Autodesk Inventor part; units mm, degrees
(part 3 of 3)
sketch "Sketch14" plane through (63, -33.9467, -18.5) normal (0, 0, -1) x (-1, 0, 0)
  line L0 (10.55, 31.8934) -> (35, 31.8934) construction
  line L1 (35, 29.5934) -> (35, 31.8934) construction
  line L2 (32.7, 27.2934) -> (35, 29.5934) construction
  line L3 (7.65, 27.2934) -> (32.7, 27.2934) construction
  line L4 (7.65, 29.4734) -> (7.65, 27.2934) construction
  line L5 (0, 29.4734) -> (7.65, 29.4734) construction
  line L6 (0, 35.2734) -> (0, 29.4734) construction
  line L7 (1.6, 35.2734) -> (0, 35.2734) construction
  line L8 (1.6, 44.1134) -> (1.6, 35.2734) construction
  line L9 (0, 44.1134) -> (1.6, 44.1134) construction
  line L10 (0, 52.9934) -> (0, 44.1134) construction
  line L11 (32.7, 52.9934) -> (0, 52.9934) construction
  line L12 (35, 50.6934) -> (32.7, 52.9934) construction
  line L13 (35, 47.8934) -> (35, 50.6934) construction
  line L14 (35, 47.8934) -> (10.55, 47.8934) construction
  line L15 (10.55, 47.8934) -> (10.55, 31.8934) construction
  circle A0 centre (10.2, 51.4934) radius 0.5 construction
  circle A1 centre (15.2, 51.4934) radius 0.5 construction
  circle A2 centre (20.2, 51.4934) radius 0.5 construction
  circle A3 centre (25.2, 51.4934) radius 0.5 construction
  circle A4 centre (10.2, 28.7934) radius 0.5 construction
  circle A5 centre (12.7, 28.7934) radius 0.5 construction
  circle A6 centre (15.2, 28.7934) radius 0.5 construction
  circle A7 centre (17.7, 28.7934) radius 0.5 construction
  circle A8 centre (20.2, 28.7934) radius 0.5 construction
  circle A9 centre (22.7, 28.7934) radius 0.5 construction
  circle A10 centre (25.2, 28.7934) radius 0.5 construction
  circle A11 centre (27.7, 28.7934) radius 0.5 construction
  circle A12 centre (27.7, 51.4934) radius 0.5 construction
  circle A13 centre (22.7, 51.4934) radius 0.5 construction
  circle A14 centre (17.7, 51.4934) radius 0.5 construction
  circle A15 centre (12.7, 51.4934) radius 0.5 construction
  line L16 (1.6, 43.4784) -> (1.6, 35.9084) construction
  line L17 (0.7, 35.9084) -> (1.6, 35.9084) construction
  line L18 (0.7, 43.4784) -> (0.7, 35.9084) construction
  line L19 (0.7, 43.4784) -> (1.6, 43.4784) construction
  line L20 (28.04, 47.3934) -> (28.04, 44.3934) construction
  line L21 (28.04, 44.3934) -> (29.74, 44.3934) construction
  line L22 (29.74, 44.3934) -> (29.74, 47.3934) construction
  line L23 (29.74, 47.3934) -> (28.04, 47.3934) construction
  line L24 (12.6, 45.8934) -> (12.6, 33.8934) construction
  line L25 (12.6, 33.8934) -> (27.7, 33.8934) construction
  line L26 (27.7, 33.8934) -> (27.7, 45.8934) construction
  line L27 (27.7, 45.8934) -> (12.6, 45.8934) construction
  line L28 (10.55, 47.8934) -> (35.5, 47.8934) construction
  line L29 (35.5, 47.8934) -> (35.5, 31.8934) construction
  line L30 (35.5, 31.8934) -> (10.55, 31.8934) construction
  line L31 (10.55, 31.8934) -> (10.55, 47.8934) construction
  line L32 (12.6, 45.8934) -> (27.7, 45.8934) construction
  line L33 (27.7, 45.8934) -> (27.7, 33.8934) construction
  line L34 (27.7, 33.8934) -> (12.6, 33.8934) construction
  line L35 (12.6, 33.8934) -> (12.6, 45.8934) construction
  line L36 (35, 29.5934) -> (35, 31.8934)
  line L37 (35.5, 31.8934) -> (35, 31.8934)
  line L38 (35.5, 31.8934) -> (35.5, 47.8934)
  line L39 (35.5, 47.8934) -> (35, 47.8934)
  line L40 (35, 47.8934) -> (35, 50.6934)
  line L41 (35, 50.6934) -> (32.7, 52.9934)
  line L42 (32.7, 52.9934) -> (0, 52.9934)
  line L43 (0, 52.9934) -> (0, 44.1134)
  line L44 (0, 44.1134) -> (0, 29.4734)
  line L45 (0, 29.4734) -> (7.65, 29.4734)
  line L46 (7.65, 29.4734) -> (7.65, 27.2934)
  line L47 (7.65, 27.2934) -> (32.7, 27.2934)
  line L48 (32.7, 27.2934) -> (35, 29.5934)
  line L49 (10.55, 47.8934) -> (35.5, 47.8934)
  line L50 (35.5, 47.8934) -> (35.5, 31.8934)
  line L51 (35.5, 31.8934) -> (10.55, 31.8934)
  line L52 (10.55, 31.8934) -> (10.55, 47.8934)
  line L53 (12.6, 45.8934) -> (27.7, 45.8934)
  line L54 (27.7, 45.8934) -> (27.7, 33.8934)
  line L55 (27.7, 33.8934) -> (12.6, 33.8934)
  line L56 (12.6, 33.8934) -> (12.6, 45.8934)
  line L57 (28.04, 47.3934) -> (29.74, 47.3934)
  line L58 (29.74, 47.3934) -> (29.74, 44.3934)
  line L59 (29.74, 44.3934) -> (28.04, 44.3934)
  line L60 (28.04, 44.3934) -> (28.04, 47.3934)
  line L61 (-0.15, 29.3234) -> (-0.15, 44.1134)
  line L62 (-0.15, 44.1134) -> (-0.15, 53.1434)
  line L63 (-0.15, 53.1434) -> (32.7621, 53.1434)
  line L64 (32.7621, 53.1434) -> (35.15, 50.7555)
  line L65 (35.15, 50.7555) -> (35.15, 48.0434)
  line L66 (35.15, 48.0434) -> (35.65, 48.0434)
  line L67 (35.65, 48.0434) -> (35.65, 31.7434)
  line L68 (35.65, 31.7434) -> (35.15, 31.7434)
  line L69 (35.15, 31.7434) -> (35.15, 29.5312)
  line L70 (35.15, 29.5312) -> (32.7621, 27.1434)
  line L71 (32.7621, 27.1434) -> (7.5, 27.1434)
  line L72 (7.5, 27.1434) -> (7.5, 29.3234)
  line L73 (7.5, 29.3234) -> (-0.15, 29.3234)
  line L74 (10.4, 31.7434) -> (10.4, 48.0434)
  line L75 (10.4, 48.0434) -> (35.65, 48.0434)
  line L76 (35.65, 48.0434) -> (35.65, 31.7434)
  line L77 (35.65, 31.7434) -> (10.4, 31.7434)
  line L78 (12.45, 46.0434) -> (27.85, 46.0434)
  line L79 (27.85, 46.0434) -> (27.85, 33.7434)
  line L80 (27.85, 33.7434) -> (12.45, 33.7434)
  line L81 (12.45, 33.7434) -> (12.45, 46.0434)
  line L82 (27.89, 44.2434) -> (27.89, 47.5434)
  line L83 (27.89, 47.5434) -> (29.89, 47.5434)
  line L84 (29.89, 47.5434) -> (29.89, 44.2434)
  line L85 (29.89, 44.2434) -> (27.89, 44.2434)
  line L86 (7.5, 27.1434) -> (-0.15, 27.1434)
  line L87 (-0.15, 27.1434) -> (-0.15, 29.3234)
  line L88 (29.2, 50.4934) -> (8.7, 50.4934)
  line L89 (8.7, 50.4934) -> (8.7, 52.7434)
  line L90 (8.7, 52.7434) -> (29.2, 52.7434)
  line L91 (29.2, 52.7434) -> (29.2, 50.4934)
  line L92 (37.9136, 28.7934) -> (37.9136, 51.4934) construction
  line L93 (0, 54.9934) -> (63, 54.9934) construction
  line L94 (37.9136, 40.1434) -> (-2.924, 40.1434) construction
  line L95 (29.2, 29.7934) -> (8.7, 29.7934)
  line L96 (8.7, 29.7934) -> (8.7, 27.5434)
  line L97 (8.7, 27.5434) -> (29.2, 27.5434)
  line L98 (29.2, 27.5434) -> (29.2, 29.7934)
  point P0 (63, 33.9467)
  point P1 (35, 48.0434)
  point P2 (35, 31.7434)
  point P3 (35.15, 48.0434)
  point P4 (35.15, 31.7434)
  dimension "d69" = 0.15
  dimension "d70" = 0.15
  dimension "d71" = 0.15
  dimension "d72" = 0.15
  dimension "d88" = 1
  dimension "d90" = 1
  dimension "d91" = 0.75
  dimension "d92" = 1
  constraints: 124 end point, 13 collinear, 9 parallel, 6 horizontal, 6 perpendicular, 4 symmetric about line, 1 midpoint, 21 other
  measures "d69" distance between parallel lines of L44 L61
  measures "d70" distance between parallel lines of L15 L74
  measures "d71" distance between parallel lines of L35 L81
  measures "d72" distance between parallel lines of L20 L82
  measures "d88" distance edge to line of A0 L89
  measures "d90" distance edge to line of A12 L91
  measures "d91" distance edge to line of A12 L90
  measures "d92" distance from line of L88 A12.centre
extrude "Extrusion12" cut sketch "Sketch14" against normal blind 13.7 contours L53 L54 L55 L56 | L78 L79 L80 L81
extrude "Extrusion13" cut sketch "Sketch14" against normal blind 11.4 contours L77 L74 L75 L40 L49 L52 L51 L36 | L36 L37 L38 L39 L40 L75 L66 L67 L68 L77 | L51 L52 L49 L39 L38 L37 | L57 L58 L59 L60 | L82 L83 L84 L85 | L88 L89 L90 L91 | L98 L97 L96 L95
extrude "Extrusion14" cut sketch "Sketch14" against normal blind 12.05 contours L57 L58 L59 L60 | L82 L83 L84 L85
extrude "Extrusion15" cut sketch "Sketch14" against normal blind 10.4 contours L48 L47 L46 L45 L44 L43 L42 L41 L40 L75 L74 L77 L36 | L36 L77 L69 L70 L71 L72 L73 L61 L62 L63 L64 L65 L75 L40 L41 L42 L43 L44 L45 L46 L47 L48 | L86 L87 L73 L72 | L88 L89 L90 L91 | L98 L97 L96 L95
sketch "Sketch16" plane through (63, -33.9467, -18.5) normal (0, 0, -1) x (-1, 0, 0)
  line L0 (52.95, 50.8534) -> (45.85, 50.8534) construction
  line L1 (45.85, 50.8534) -> (45.85, 30.8534) construction
  line L2 (45.85, 30.8534) -> (52.95, 30.8534) construction
  line L3 (52.95, 30.8534) -> (52.95, 50.8534) construction
  line L4 (54, 31.7134) -> (44.8, 31.7134) construction
  line L5 (44.8, 31.7134) -> (44.8, 49.9934) construction
  line L6 (44.8, 49.9934) -> (54, 49.9934) construction
  line L7 (54, 49.9934) -> (54, 31.7134) construction
  line L8 (53.1, 30.7034) -> (45.7, 30.7034)
  line L9 (45.7, 30.7034) -> (45.7, 51.0034)
  line L10 (45.7, 51.0034) -> (53.1, 51.0034)
  line L11 (53.1, 51.0034) -> (53.1, 30.7034)
  line L12 (55, 30.7134) -> (43.8, 30.7134)
  line L13 (43.8, 30.7134) -> (43.8, 50.9934)
  line L14 (43.8, 50.9934) -> (55, 50.9934)
  line L15 (55, 50.9934) -> (55, 30.7134)
  point P0 (63, 33.9467)
  dimension "d93" = 0.15
  dimension "d94" = 1
  constraints: 32 end point, 8 parallel, 4 perpendicular, 2 horizontal, 10 other
  measures "d93" distance between parallel lines of L2 L8
  measures "d94" distance between parallel lines of L7 L15
extrude "Extrusion17" cut sketch "Sketch16" against normal blind 13.7 contours L8 L9 L12 L11 | L12 L9 L14 L11 | L14 L9 L10 L11
extrude "Extrusion18" cut sketch "Sketch16" against normal blind 12.3 contours L12 L9 L14 L11 | L11 L14 L15 L12 | L12 L13 L14 L9
sketch "Sketch15" plane through (63, -33.9467, -18.5) normal (0, 0, -1) x (-1, 0, 0)
  line L0 (38.15, 22.15) -> (38.15, 5.85) projected
  line L1 (38.15, 5.85) -> (24.85, 5.85)
  line L2 (24.85, 5.85) -> (24.85, 30.7134)
  line L3 (38.15, 30.7134) -> (38.15, 5.85)
  line L4 (24.85, 5.85) -> (24.85, 22.15) projected
  line L5 (24.85, 30.7134) -> (55, 30.7134)
  line L6 (55, 30.7134) -> (55, 40.7134)
  line L7 (55, 40.7134) -> (24.85, 40.7134)
  line L8 (24.85, 40.7134) -> (24.85, 30.7134)
  line L9 (45.7, 30.7134) -> (43.8, 30.7134) projected
  line L10 (55, 50.9934) -> (55, 30.7134) projected
  point P0 (63, 33.9467)
  point P1 (35.5, 37.3828)
  point P2 (38.15, 22.15)
  dimension "d99" = 10
  constraints: 14 end point, 3 collinear, 3 parallel, 3 perpendicular, 2 horizontal, 1 point on line
  measures "d99" distance between parallel lines of L5 L7
extrude "Extrusion16" cut sketch "Sketch15" against normal blind 5
chamfer "Chamfer2" distance 2 angle 45 10 edges at (19.2, 1.7667, -13.5) (27.35, 2.2817, -13.5) (27.6, -2.2033, -13.5) (27.85, -3.3094, -13.5) (29.0439, -5.6094, -13.5) (34.1939, -6.8033, -13.5) (24.85, -3.2333, -16) (38.15, -6.8033, -16) (27.35, 6.7667, -16) (19.2, 6.7667, -16)
body "Solid3"
